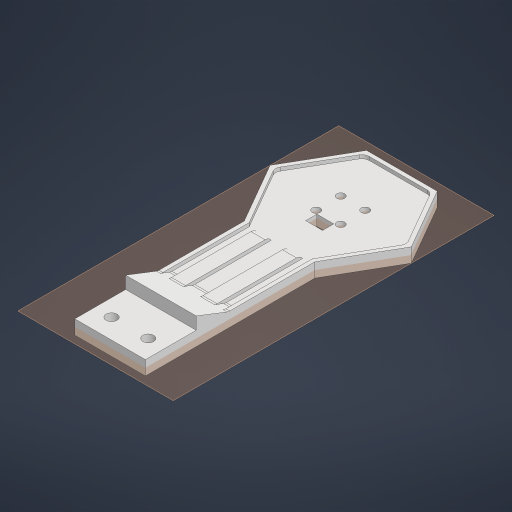
# Autodesk Inventor part: Arm
Saved by Autodesk Inventor 2023 (Build 270158000, 158)
## iProperties
Created: 2023-01-21
Part Number: Arm
Material: Generic
Document SubType Name: Modeling
Designer: Michael
Density: 1 g/cm^3
Appearance: Default
Author: Michael
Autodesk Inventor part; units mm, degrees
ref_plane "YZ Plane" through (0, 0, 0) normal (1, 0, 0) x (0, 1, 0)
ref_plane "XZ Plane" through (0, 0, 0) normal (0, 1, 0) x (-1, 0, 0)
ref_plane "XY Plane" through (0, 0, 0) normal (0, 0, 1) x (1, 0, 0)
sketch "Sketch1" plane through (0, 0, 0) normal (0, 1, 0) x (-1, 0, 0)
  line L0 (0, 0) -> (31.75, 0)
  line L1 (31.75, 0) -> (31.75, -76.2)
  line L2 (31.75, -76.2) -> (0, -76.2)
  line L3 (0, -76.2) -> (0, 0)
  line L4 (31.75, -131.1926) -> (0, -131.1926)
  line L5 (0, -131.1926) -> (-15.875, -103.6963)
  line L6 (-15.875, -103.6963) -> (0, -76.2)
  line L7 (0, -76.2) -> (31.75, -76.2)
  line L8 (31.75, -76.2) -> (47.625, -103.6963)
  line L9 (47.625, -103.6963) -> (31.75, -131.1926)
  line L10 (10.3741, -98.1972) -> (21.3741, -98.1972)
  line L11 (21.3741, -98.1972) -> (21.3741, -109.1972)
  line L12 (21.3741, -109.1972) -> (10.3741, -109.1972)
  line L13 (10.3741, -109.1972) -> (10.3741, -98.1972)
  circle A0 centre (21.3741, -98.1972) radius 1.8034
  circle A1 centre (21.3741, -109.1972) radius 1.8034
  circle A2 centre (10.3741, -109.1972) radius 1.8034
  circle A3 centre (10.3741, -98.1972) radius 1.8034
  line L14 (15.875, -131.1926) -> (15.875, -76.2)
  line L15 (47.625, -103.6963) -> (-15.875, -103.6963)
  line L16 (19.685, -91.7208) -> (12.065, -91.7208)
  line L17 (12.065, -91.7208) -> (12.065, -96.8008)
  line L18 (12.065, -96.8008) -> (19.685, -96.8008)
  line L19 (19.685, -96.8008) -> (19.685, -91.7208)
  point P0 (15.875, -103.6963)
  point P1 (15.8741, -98.1972)
  point P2 (31.75, -76.2)
  point P3 (0, -76.2)
  dimension "d0" = 31.75
  dimension "d1" = 76.2
  dimension "d65" = 31.75
  dimension "d66" = 11
  dimension "d67" = 11
  dimension "d68" = 5.4991
  dimension "d69" = 5.4991
  dimension "d70" = 3.6068
  dimension "d71" = 3.6068
  dimension "d72" = 3.6068
  dimension "d73" = 3.6068
  dimension "d94" = 5.08
  dimension "d96" = -1.6909
  dimension "d97" = 7.62
  dimension "d98" = 3.81
  constraints: 40 end point, 7 parallel, 4 centre point, 4 coincident, 4 horizontal, 4 midpoint, 3 perpendicular, 1 vertical, 13 other
  measures "d0" distance of L1.end L2.end
  measures "d1" distance of L0.end L1.end
  measures "d65" distance of L6.end L7.end
  measures "d66" distance of L10.start L10.end
  measures "d67" distance of L10.end L11.end
  measures "d68" distance from line of L11 point (15.875, -103.696)
  measures "d69" distance of point (15.874, -98.197) point (15.875, -103.696)
  measures "d70" diameter of A0
  measures "d71" diameter of A1
  measures "d72" diameter of A2
  measures "d73" diameter of A3
  measures "d94" distance of L17.end L16.end
  measures "d96" distance from line of A3.centre L17
  measures "d97" distance of L16.start L16.end
  measures "d98" distance between parallel lines of L17 L14
extrude "Extrusion1" add sketch "Sketch1" along normal blind 6.35 contours L0 L1 L2 L3 | L2 L14 L16 L17 L18 L10 A3 L13 L15 L6 | L8 L15 L11 A0 L10 L14 L18 L19 L16 L2 | L15 L13 A2 L12 L14 L4 L5 | L9 L4 L14 L12 A1 L11 L15 | L15 L14 L12 A2 L13 | L13 A3 L10 L14 L15 | L15 L14 L10 A0 L11 | L11 A1 L12 L14 L15
sketch "Sketch4" plane through (0, 6.35, 0) normal (0, 1, 0) x (1, 0, 0)
  circle A0 centre (-7.62, 8.89) radius 2.4765
  line L0 (-31.75, 0) -> (0, 0) projected
  line L1 (0, 0) -> (0, 76.2) projected
  circle A1 centre (-24.13, 8.89) radius 2.4765
  line L2 (-31.75, 76.2) -> (-31.75, 0) projected
  point P0 (0, 127)
  point P1 (-31.75, 127)
  dimension "d11" = 4.953
  dimension "d12" = 8.89
  dimension "d13" = 7.62
  dimension "d14" = 4.953
  dimension "d15" = 8.89
  dimension "d16" = 7.62
  constraints: 2 centre point
  measures "d11" diameter of A0
  measures "d12" distance from line of L0 A0.centre
  measures "d13" distance from line of A0.centre L1
  measures "d14" diameter of A1
  measures "d15" distance from line of L0 A1.centre
  measures "d16" distance from line of L2 A1.centre
extrude "Extrusion4" cut sketch "Sketch4" against normal blind 36.5125
sketch "Sketch8" plane through (0, 6.35, 0) normal (0, 1, 0) x (1, 0, 0)
  circle A0 centre (-10.3741, 98.1972) radius 1.8034 projected
  circle A1 centre (-10.3741, 109.1972) radius 1.8034 projected
  circle A2 centre (-21.3741, 109.1972) radius 1.8034 projected
  circle A3 centre (-21.3741, 98.1972) radius 1.8034 projected
  line L0 (0, 0) -> (0, 76.2) projected
  line L1 (0, 76.2) -> (15.875, 103.6963) projected
  line L2 (15.875, 103.6963) -> (0, 131.1926) projected
  line L3 (0, 131.1926) -> (-31.75, 131.1926) projected
  line L4 (-31.75, 131.1926) -> (-47.625, 103.6963) projected
  line L5 (-47.625, 103.6963) -> (-31.75, 76.2) projected
  line L6 (-31.75, 76.2) -> (-31.75, 0) projected
  line L7 (-30.0159, 27.1341) -> (-1.7341, 27.1341)
  line L8 (-1.7341, 27.1341) -> (-1.7341, 76.6646)
  line L9 (-1.7341, 76.6646) -> (13.8726, 103.6963)
  line L10 (13.8726, 103.6963) -> (-1.0012, 129.4585)
  line L11 (-1.0012, 129.4585) -> (-30.7488, 129.4585)
  line L12 (-30.7488, 129.4585) -> (-45.6226, 103.6963)
  line L13 (-45.6226, 103.6963) -> (-30.0159, 76.6646)
  line L14 (-30.0159, 76.6646) -> (-30.0159, 27.1341)
  line L15 (-31.75, 0) -> (0, 0) projected
  constraints: 16 end point, 6 other
extrude "Extrusion7" cut sketch "Sketch8" against normal blind 1.5875 contours L14 L13 L12 L11 L10 L9 L8 L7
sketch "Sketch9" plane through (-1.7341, 6.35, -27.1341) normal (0, 0, -1) x (-1, 0, 0)
  line L0 (0, 0) -> (28.2818, 0) projected
  line L1 (0, 0) -> (0, -1.5875) projected
  line L2 (0, -1.5875) -> (28.2818, -1.5875) projected
  line L3 (28.2818, 0) -> (28.2818, -1.5875) projected
  line L4 (30.0159, 0) -> (-1.7341, 0) projected
  line L5 (14.1409, 0) -> (14.1409, -1.5875)
  line L6 (21.2148, 0) -> (24.3898, 0)
  line L7 (-1.7341, -3.175) -> (30.0159, -3.175) projected
  line L8 (21.2148, 0) -> (18.0398, 0)
  line L9 (18.0398, 0) -> (18.0398, -1.5875)
  line L10 (24.3898, 0) -> (24.3898, -1.5875)
  line L11 (28.2818, 0) -> (0, 0)
  line L12 (-1.7341, 0) -> (30.0159, 0)
  line L13 (7.067, 0) -> (3.892, 0)
  line L14 (7.067, 0) -> (10.242, 0)
  line L15 (10.242, 0) -> (10.242, -1.5875)
  line L16 (3.892, 0) -> (3.892, -1.5875)
  point P0 (-1.7341, -6.35)
  point P1 (14.1409, -0.7937)
  point P2 (3.892, 0)
  point P3 (3.892, -1.5875)
  point P4 (10.242, 0)
  dimension "d79" = 7.0739
  dimension "d80" = 3.175
  dimension "d82" = 3.175
  constraints: 22 end point, 9 symmetric about line, 4 point on line, 3 midpoint, 2 perpendicular, 1 collinear, 1 horizontal
  measures "d79" horizontal distance of point (14.141, -0.794) L6.start
  measures "d80" distance of L6.start L6.end
  measures "d82" distance of L6.start L8.end
extrude "Extrusion8" add sketch "Sketch9" along normal blind 49.2125 contours L0 L15 L2 L16 | L0 L10 L2 L9
fillet "Fillet2" radius 3.175 2 edges at (-8.8011, 6.35, -76.3466) (-22.9489, 6.35, -76.3466)
fillet "Fillet4" radius 3.175 4 edges at (-45.6226, 5.5562, -103.6963) (13.8726, 5.5562, -103.6963) (-30.7488, 5.5562, -129.4585) (-1.0012, 5.5562, -129.4585)
ref_plane "Work Plane1" through (0, 3.175, 0) normal (0, 1, 0) x (1, 0, 0)
sketch "Sketch11" plane through (0, 3.175, 0) normal (0, 1, 0) x (1, 0, 0)
  line L0 (-0.0667, 22.8993) -> (-31.8167, 22.8612)
  line L1 (0, 25.4) -> (0, 0) projected
  line L2 (-31.75, 25.4) -> (0, 25.4) projected
  line L3 (-31.75, 0) -> (-31.75, 25.4) projected
  line L4 (0, 25.4) -> (-31.75, 25.4)
  line L5 (-31.75, 25.4) -> (-31.75, 22.8613)
  line L6 (-31.75, 22.8613) -> (0, 22.8613)
  line L7 (0, 22.8613) -> (0, 25.4)
  constraints: 10 end point, 2 parallel, 2 point on line, 1 horizontal, 1 perpendicular, 3 other
extrude "Extrusion9" add sketch "Sketch11" along normal blind 3.175
sketch "Sketch13" plane through (0, 6.35, 0) normal (0, 1, 0) x (1, 0, 0)
  line L0 (-1.1058, 21.2778) -> (-31.081, 21.2778)
  line L1 (-31.081, 21.2778) -> (-31.081, 31.4378)
  line L2 (-31.081, 31.4378) -> (-1.1058, 31.4378)
  line L3 (-1.1058, 31.4378) -> (-1.1058, 21.2778)
  point P0 (0, 0)
  dimension "d99" = 10.16
  constraints: 8 end point, 2 parallel, 1 horizontal, 1 perpendicular
  measures "d99" distance of L0.end L1.end
extrude "Extrusion11" add sketch "Sketch13" against normal blind 3.175
sketch "Sketch14" plane through (-31.75, 0, -76.2) normal (-1, 0, 0) x (0, 0, 1)
  line L0 (44.7622, 6.35) -> (53.3387, 6.35)
  line L1 (0, 6.35) -> (76.2, 6.35) projected
  line L2 (44.7622, 4.7625) -> (-0.1466, 4.7625) projected
  line L3 (44.7622, 6.35) -> (2.603, 6.35) projected
  line L4 (53.3387, 6.35) -> (53.3387, 4.7625)
  line L5 (53.3387, 4.7625) -> (34.8482, 4.7625)
  line L6 (53.3387, 6.35) -> (53.3387, 11.938)
  line L7 (53.3387, 11.938) -> (34.8482, 4.7625)
  point P0 (76.2, 0)
  dimension "d107" = 5.588
  constraints: 10 end point, 2 perpendicular, 2 point on line, 1 collinear, 1 vertical, 1 other
  measures "d107" distance of L0.end L6.end
extrude "Extrusion12" add sketch "Sketch14" against normal blind 31.75
fillet "Fillet9" radius 3.175 7 edges at (-0.867, 6.35, -37.261) (-8.8011, 6.35, -37.261) (-22.9489, 6.35, -37.261) (-30.883, 6.35, -37.261) (-15.875, 4.7625, -41.3518) (-28.0699, 4.7625, -41.3518) (-3.6801, 4.7625, -41.3518)
body "Solid1"
